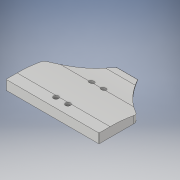
# Autodesk Inventor part: Lump v2
Saved by Autodesk Inventor 2019 (Build 230136000, 136)
## iProperties
Created: 2019-01-07
Part Number: Lump v2
Material: Generic
Document SubType Name: Modeling
Designer: ashle
Density: 1 g/cm^3
Appearance: Default
Author: ashle
Autodesk Inventor part; units mm, degrees
ref_plane "YZ Plane" through (0, 0, 0) normal (1, 0, 0) x (0, 1, 0)
ref_plane "XZ Plane" through (0, 0, 0) normal (0, 1, 0) x (-1, 0, 0)
sketch "Sketch1" plane through (0, 0, 0) normal (0, 1, 0) x (-1, 0, 0)
  line L0 (13.5, -50.8) -> (-13.5, -50.8)
  line L1 (-13.5, -50.8) -> (-13.5, 0)
  line L2 (13.5, 0) -> (13.5, -50.8)
  line L3 (-62.5, 0) -> (-62.5, 50.8)
  line L4 (-62.5, 50.8) -> (62.5, 50.8)
  line L5 (62.5, 50.8) -> (62.5, 0)
  line L6 (62.5, 0) -> (13.5, 0)
  line L7 (-13.5, 0) -> (-62.5, 0)
  point P0 (0, 0)
  dimension "d1" = 27
  dimension "d2" = 13.5
  dimension "d7" = 125
  dimension "d8" = 62.5
  dimension "d10" = 50.8
  dimension "d11" = 50.8
  dimension "d12" = 50.8
  dimension "d13" = 50.8
  constraints: 16 end point, 4 parallel, 3 horizontal, 3 perpendicular
  measures "d1" distance between parallel lines of L1 L2
  measures "d2" distance from line of L1 point (0, 0)
  measures "d7" distance between parallel lines of L3 L5
  measures "d8" distance from line of point (0, 0) L3
  measures "d10" distance between parallel lines of L7 L4
  measures "d11" distance between parallel lines of L0 L7
  measures "d12" distance between parallel lines of L0 L6
  measures "d13" distance from line of point (0, 0) L0
extrude "Extrusion1" add sketch "Sketch1" along normal blind 12.7
fillet "Fillet3" radius 140 2 edges at (13.5, 6.35, 0) (-13.5, 6.35, 0)
sketch "Sketch3" plane through (0, 12.7, 0) normal (0, 1, 0) x (1, 0, 0)
  line L0 (-38.1, 25.4) -> (38.1, 25.4)
  line L1 (38.1, 25.4) -> (38.1, 50.8)
  line L2 (38.1, 50.8) -> (-38.1, 50.8)
  line L3 (-38.1, 50.8) -> (-38.1, 25.4)
  point P0 (0, 0)
  dimension "d21" = 25.4
  dimension "d22" = 25.4
  dimension "d24" = 38.1
  dimension "d26" = 38.1
  constraints: 8 end point, 2 parallel, 1 horizontal, 1 perpendicular
  measures "d21" distance from line of point (0, 0) L0
  measures "d22" distance between parallel lines of L0 L2
  measures "d24" distance from line of point (0, 0) L3
  measures "d26" distance from line of point (0, 0) L1
extrude "Extrusion2" cut sketch "Sketch3" against normal blind 11.43
fillet "Fillet4" radius 170 1 edges at (0, 12.7, -25.4)
fillet "Fillet5" radius 150 1 edges at (0, 1.27, -25.4)
fillet "Fillet6" radius 60 1 edges at (0, 1.27, -50.8)
fillet "Fillet7" radius 7 2 edges at (62.5, 4.435, 0) (-62.5, 4.435, 0)
fillet "Fillet8" radius 1 2 edges at (62.5, 6.35, 50.8) (-62.5, 6.35, 50.8)
fillet "Fillet10" radius 0.1 10 edges at (33.4466, 0, -23.6269) (61.651, 0, 0.5217) (62.5, 0, 26.8316) (62.2071, 0, 50.5071) (0, 0, 50.8) (-62.2071, 0, 50.5071) (-62.5, 0, 26.8316) (-61.651, 0, 0.5217) (-33.4466, 0, -23.6269) (0, 0, -50.8)
sketch "Sketch4" plane through (0, 0, 0) normal (0, -1, 0) x (1, 0, 0)
  circle A0 centre (8, -9.9127) radius 2.15
  circle A1 centre (-8, -9.9127) radius 2.15
  line L0 (8, -9.9127) -> (-8, -9.9127) construction
  line L1 (-61.5, 50.7) -> (61.5, 50.7) construction
  line L2 (13.8883, -49.9127) -> (-13.8883, -49.9127) construction
  circle A2 centre (8, 38.0873) radius 2.15
  circle A3 centre (-8, 38.0873) radius 2.15
  line L3 (8, 38.0873) -> (-8, 38.0873) construction
  line L4 (-8, 38.0873) -> (-8, -9.9127) construction
  line L5 (8, 38.0873) -> (8, -9.9127) construction
  line L6 (-62.4, 3.8631) -> (-62.4, 49.8) construction
  point P0 (0, 0)
  point P1 (11.5501, -49.9127)
  point P2 (-11.5501, -49.9127)
  dimension "d36" = 4.3
  dimension "d37" = 4.3
  dimension "d38" = 16
  dimension "d39" = 40
  dimension "d40" = 3.5501
  dimension "d41" = 23.1002
  dimension "d42" = 4.3
  dimension "d43" = 4.3
  dimension "d44" = 16
  dimension "d45" = 48
  constraints: 8 end point, 4 centre point, 3 parallel
  measures "d36" diameter of A0
  measures "d37" diameter of A1
  measures "d38" distance of L0.end L0.start
  measures "d39" distance between parallel lines of L2 L0
  measures "d40" horizontal distance of point (11.55, -49.913) L0.start
  measures "d41" distance of point (11.55, -49.913) point (-11.55, -49.913)
  measures "d42" diameter of A2
  measures "d43" diameter of A3
  measures "d44" distance of L3.start L3.end
  measures "d45" distance between parallel lines of L3 L0
extrude "Extrusion3" cut sketch "Sketch4" against normal blind 12.7
sketch "Sketch5" plane through (0, 12.7, 0) normal (0, 1, 0) x (1, 0, 0)
  circle A0 centre (8, -38.0873) radius 2.15 projected
  circle A1 centre (8, -38.0873) radius 3.25
  circle A2 centre (-8, -38.0873) radius 2.15 projected
  circle A3 centre (-8, -38.0873) radius 3.25
  point P0 (0, 0)
  dimension "d51" = 6.5
  dimension "d52" = 6.5
  constraints: 2 centre point, 2 coincident
  measures "d51" diameter of A3
  measures "d52" diameter of A1
extrude "Extrusion4" cut sketch "Sketch5" against normal blind 10.7
ref_plane "Work Plane1" through (0, 7, 0) normal (0, -1, 0) x (1, 0, 0)
sketch "Sketch6" plane through (0, 7, 0) normal (0, -1, 0) x (1, 0, 0)
  circle A0 centre (-8, -9.9127) radius 2.15 projected
  circle A1 centre (-8, -9.9127) radius 3.25
  circle A2 centre (8, -9.9127) radius 2.15 projected
  circle A3 centre (8, -9.9127) radius 3.25
  point P0 (0, 0)
  dimension "d53" = 6.5
  dimension "d54" = 6.5
  constraints: 2 centre point, 2 coincident
  measures "d53" diameter of A1
  measures "d54" diameter of A3
extrude "Extrusion5" cut sketch "Sketch6" along normal blind 5
sketch "Sketch7" plane through (0, 7, 0) normal (0, -1, 0) x (1, 0, 0)
  arc A0 (10.4432, -7.7696) -> (5.5568, -7.7696) centre (8, -9.9127) ccw construction
  arc A1 (8.1714, -7.7696) -> (7.8286, -7.7696) centre (8, -9.9127) ccw construction
  circle A2 centre (8, -9.9127) radius 3.25
  line L0 (0, -11.645) -> (0, -4.6146) construction
  line L1 (-10.4432, -7.7696) -> (-8.1714, -7.7696) construction
  arc A3 (-5.5568, -7.7696) -> (-10.4432, -7.7696) centre (-8, -9.9127) ccw construction
  line L2 (-7.8286, -7.7696) -> (-5.5568, -7.7696) construction
  arc A4 (-7.8286, -7.7696) -> (-8.1714, -7.7696) centre (-8, -9.9127) ccw construction
  circle A5 centre (-8, -9.9127) radius 3.25
  point P0 (0, 0)
  constraints: 7 symmetric about line, 6 end point, 4 centre point, 4 point on circle, 2 coincident, 1 vertical, 3 other
extrude "Extrusion6" cut sketch "Sketch7" against normal blind 10
equation "\"d2\" = 0.5 * d1"
equation "\"d8\" = 0.5 * d7"
equation "\"d10\" = d4"
equation "\"d37\" = d36"
equation "\"d42\" = d36"
equation "\"d43\" = d36"
equation "\"d52\" = d51"
equation "\"d54\" = d53"
equation "\"d4\" = 0.5 * d3"
equation "\"d5\" = d4"
equation "\"d3\" = 101.6"
body "Solid1"
